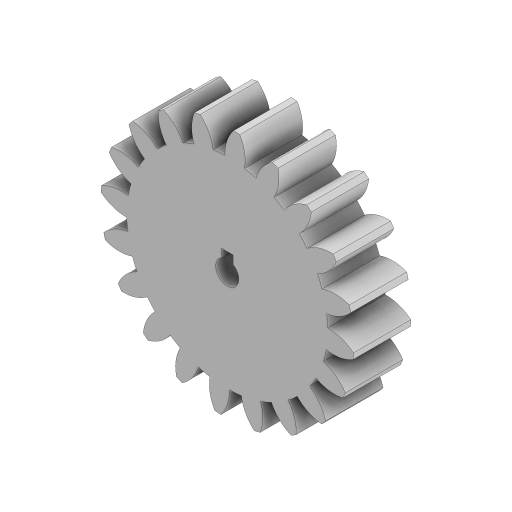
# Autodesk Inventor part: ENGRANE MOTRIZ DE CAJA
Saved by Autodesk Inventor 2024 (Build 280153000, 153)
## iProperties
Created: 2024-06-16
Part Number: ENGRANE MOTRIZ DE CAJA
Material: Generic
Document SubType Name: Modeling
Designer: Jhuliams
Density: 1 g/cm^3
Appearance: Default
Author: Jhuliams
Autodesk Inventor part; units mm, degrees
ref_plane "YZ Plane" through (0, 0, 0) normal (1, 0, 0) x (0, 1, 0)
ref_plane "XZ Plane" through (0, 0, 0) normal (0, 1, 0) x (-1, 0, 0)
ref_plane "XY Plane" through (0, 0, 0) normal (0, 0, 1) x (1, 0, 0)
sketch "Sketch1" plane through (0, 0, 0) normal (0, 0, 1) x (1, 0, 0)
  arc A0 (32.8389, -3.2565) -> (32.9574, -1.6756) centre (0, 0) ccw
  circle A1 centre (0, 0) radius 26.25
  line L0 (0, 0) -> (42.2346, 0) construction
  line L1 (0, 0) -> (37.3319, 0) construction
  arc A2 (32.9574, -1.6756) -> (26.2428, 0.6158) centre (26.4907, -9.6418) ccw
  line L2 (0, 0) -> (41.4252, 0) construction
  arc A3 (25.8577, -4.5212) -> (32.8389, -3.2565) centre (27.632, 5.5848) ccw
  arc A4 (32.238, 7.0507) -> (31.8622, 8.5908) centre (0, 0) ccw
  arc A5 (31.8622, 8.5908) -> (24.7681, 8.6951) centre (28.1736, -0.9838) ccw
  arc A6 (25.9893, 3.6905) -> (32.238, 7.0507) centre (24.5538, 13.8502) ccw
  arc A7 (28.4814, 16.6677) -> (27.648, 18.0163) centre (0, 0) ccw
  arc A8 (27.648, 18.0163) -> (20.8689, 15.9233) centre (27.0987, 7.7704) ccw
  arc A9 (23.5768, 11.541) -> (28.4814, 16.6677) centre (19.0721, 20.7599) ccw
  arc A10 (21.9368, 24.6531) -> (20.7275, 25.6782) centre (0, 0) ccw
  arc A11 (20.7275, 25.6782) -> (14.9269, 21.5928) centre (23.3712, 15.7641) ccw
  arc A12 (18.8565, 18.2618) -> (21.9368, 24.6531) centre (11.7235, 25.6375) ccw
  arc A13 (13.2449, 30.2254) -> (11.778, 30.8266) centre (0, 0) ccw
  arc A14 (11.778, 30.8266) -> (7.5238, 25.1487) centre (17.356, 22.2146) ccw
  arc A15 (12.2904, 23.195) -> (13.2449, 30.2254) centre (3.2273, 28.0054) ccw
  arc A16 (3.2565, 32.8389) -> (1.6756, 32.9574) centre (0, 0) ccw
  arc A17 (1.6756, 32.9574) -> (-0.6158, 26.2428) centre (9.6418, 26.4907) ccw
  arc A18 (4.5212, 25.8577) -> (3.2565, 32.8389) centre (-5.5848, 27.632) ccw
  arc A19 (-7.0507, 32.238) -> (-8.5908, 31.8622) centre (0, 0) ccw
  arc A20 (-8.5908, 31.8622) -> (-8.6951, 24.7681) centre (0.9838, 28.1736) ccw
  arc A21 (-3.6905, 25.9893) -> (-7.0507, 32.238) centre (-13.8502, 24.5538) ccw
  arc A22 (-16.6677, 28.4814) -> (-18.0163, 27.648) centre (0, 0) ccw
  arc A23 (-18.0163, 27.648) -> (-15.9233, 20.8689) centre (-7.7704, 27.0987) ccw
  arc A24 (-11.541, 23.5768) -> (-16.6677, 28.4814) centre (-20.7599, 19.0721) ccw
  arc A25 (-24.6531, 21.9368) -> (-25.6782, 20.7275) centre (0, 0) ccw
  arc A26 (-25.6782, 20.7275) -> (-21.5928, 14.9269) centre (-15.7641, 23.3712) ccw
  arc A27 (-18.2618, 18.8565) -> (-24.6531, 21.9368) centre (-25.6375, 11.7235) ccw
  arc A28 (-30.2254, 13.2449) -> (-30.8266, 11.778) centre (0, 0) ccw
  arc A29 (-30.8266, 11.778) -> (-25.1487, 7.5238) centre (-22.2146, 17.356) ccw
  arc A30 (-23.195, 12.2904) -> (-30.2254, 13.2449) centre (-28.0054, 3.2273) ccw
  arc A31 (-32.8389, 3.2565) -> (-32.9574, 1.6756) centre (0, 0) ccw
  arc A32 (-32.9574, 1.6756) -> (-26.2428, -0.6158) centre (-26.4907, 9.6418) ccw
  arc A33 (-25.8577, 4.5212) -> (-32.8389, 3.2565) centre (-27.632, -5.5848) ccw
  arc A34 (-32.238, -7.0507) -> (-31.8622, -8.5908) centre (0, 0) ccw
  arc A35 (-31.8622, -8.5908) -> (-24.7681, -8.6951) centre (-28.1736, 0.9838) ccw
  arc A36 (-25.9893, -3.6905) -> (-32.238, -7.0507) centre (-24.5538, -13.8502) ccw
  arc A37 (-28.4814, -16.6677) -> (-27.648, -18.0163) centre (0, 0) ccw
  arc A38 (-27.648, -18.0163) -> (-20.8689, -15.9233) centre (-27.0987, -7.7704) ccw
  arc A39 (-23.5768, -11.541) -> (-28.4814, -16.6677) centre (-19.0721, -20.7599) ccw
  arc A40 (-21.9368, -24.6531) -> (-20.7275, -25.6782) centre (0, 0) ccw
  arc A41 (-20.7275, -25.6782) -> (-14.9269, -21.5928) centre (-23.3712, -15.7641) ccw
  arc A42 (-18.8565, -18.2618) -> (-21.9368, -24.6531) centre (-11.7235, -25.6375) ccw
  arc A43 (-13.2449, -30.2254) -> (-11.778, -30.8266) centre (0, 0) ccw
  arc A44 (-11.778, -30.8266) -> (-7.5238, -25.1487) centre (-17.356, -22.2146) ccw
  arc A45 (-12.2904, -23.195) -> (-13.2449, -30.2254) centre (-3.2273, -28.0054) ccw
  arc A46 (-3.2565, -32.8389) -> (-1.6756, -32.9574) centre (0, 0) ccw
  arc A47 (-1.6756, -32.9574) -> (0.6158, -26.2428) centre (-9.6418, -26.4907) ccw
  arc A48 (-4.5212, -25.8577) -> (-3.2565, -32.8389) centre (5.5848, -27.632) ccw
  arc A49 (7.0507, -32.238) -> (8.5908, -31.8622) centre (0, 0) ccw
  arc A50 (8.5908, -31.8622) -> (8.6951, -24.7681) centre (-0.9838, -28.1736) ccw
  arc A51 (3.6905, -25.9893) -> (7.0507, -32.238) centre (13.8502, -24.5538) ccw
  arc A52 (16.6677, -28.4814) -> (18.0163, -27.648) centre (0, 0) ccw
  arc A53 (18.0163, -27.648) -> (15.9233, -20.8689) centre (7.7704, -27.0987) ccw
  arc A54 (11.541, -23.5768) -> (16.6677, -28.4814) centre (20.7599, -19.0721) ccw
  arc A55 (24.6531, -21.9368) -> (25.6782, -20.7275) centre (0, 0) ccw
  arc A56 (25.6782, -20.7275) -> (21.5928, -14.9269) centre (15.7641, -23.3712) ccw
  arc A57 (18.2618, -18.8565) -> (24.6531, -21.9368) centre (25.6375, -11.7235) ccw
  arc A58 (30.2254, -13.2449) -> (30.8266, -11.778) centre (0, 0) ccw
  arc A59 (30.8266, -11.778) -> (25.1487, -7.5238) centre (22.2146, -17.356) ccw
  arc A60 (23.195, -12.2904) -> (30.2254, -13.2449) centre (28.0054, -3.2273) ccw
  point P0 (35.5048, 11.5362)
  point P1 (30.2022, 21.9432)
  point P2 (21.9432, 30.2022)
  point P3 (11.5362, 35.5048)
  point P4 (0, 37.3319)
  point P5 (-11.5362, 35.5048)
  point P6 (-21.9432, 30.2022)
  point P7 (-30.2022, 21.9432)
  point P8 (-35.5048, 11.5362)
  point P9 (-37.3319, 0)
  point P10 (-35.5048, -11.5362)
  point P11 (-30.2022, -21.9432)
  point P12 (-21.9432, -30.2022)
  point P13 (-11.5362, -35.5048)
  point P14 (0, -37.3319)
  point P15 (11.5362, -35.5048)
  point P16 (21.9432, -30.2022)
  point P17 (30.2022, -21.9432)
  point P18 (35.5048, -11.5362)
  point P19 (-14.9269, -21.5928)
  point P20 (-12.2904, -23.195)
  point P21 (-7.5238, -25.1487)
  point P22 (0.6158, -26.2428)
  point P23 (3.6905, -25.9893)
  point P24 (18.2618, -18.8565)
  point P25 (21.5928, -14.9269)
  point P26 (23.195, -12.2904)
  point P27 (25.1487, -7.5238)
  point P28 (25.9893, 3.6905)
  point P29 (20.8689, 15.9233)
  point P30 (18.8565, 18.2618)
  point P31 (14.9269, 21.5928)
  point P32 (7.5238, 25.1487)
  point P33 (-0.6158, 26.2428)
  point P34 (-3.6905, 25.9893)
  point P35 (-15.9233, 20.8689)
  point P36 (-18.2618, 18.8565)
  point P37 (-21.5928, 14.9269)
  point P38 (-23.195, 12.2904)
  point P39 (-25.1487, 7.5238)
  point P40 (-26.2428, -0.6158)
  point P41 (-24.7681, -8.6951)
  point P42 (-20.8689, -15.9233)
  point P43 (-18.8565, -18.2618)
  dimension "d2" = 52.5
  dimension "d1" = 66
  dimension "d13" = 360
  constraints: 120 point on circle, 60 centre point, 6 end point, 3 horizontal, 2 coincident, 224 other
  measures "d1" diameter of A0
extrude "Extrusion1" add sketch "Sketch1" along normal blind 15
sketch "Sketch2" plane through (0, 0, 15) normal (0, 0, 1) x (1, 0, 0)
  circle A0 centre (0, 0) radius 3
  line L0 (-1.5, 4.75) -> (1.5, 4.75)
  line L1 (1.5, 4.75) -> (1.5, -4.75)
  line L2 (1.5, -4.75) -> (-1.5, -4.75)
  line L3 (-1.5, -4.75) -> (-1.5, 4.75)
  line L4 (-1.5, 4.75) -> (1.5, -4.75) construction
  line L5 (1.5, 4.75) -> (-1.5, -4.75) construction
  point P0 (-1.5, 2.5981)
  point P1 (1.5, 2.5981)
  dimension "d17" = 6
  dimension "d18" = 3
  dimension "d19" = 9.5
  constraints: 12 end point, 2 midpoint, 2 parallel, 1 centre point, 1 coincident, 1 horizontal, 1 perpendicular
  measures "d17" diameter of A0
  measures "d18" distance of L1.end L2.end
  measures "d19" distance of L0.end L1.end
extrude "Extrusion2" cut sketch "Sketch2" against normal blind 15 contours A0 L1 | L1 A0 L3 | A0 L3 L0 L1 | L3 A0
body "Solid1"
